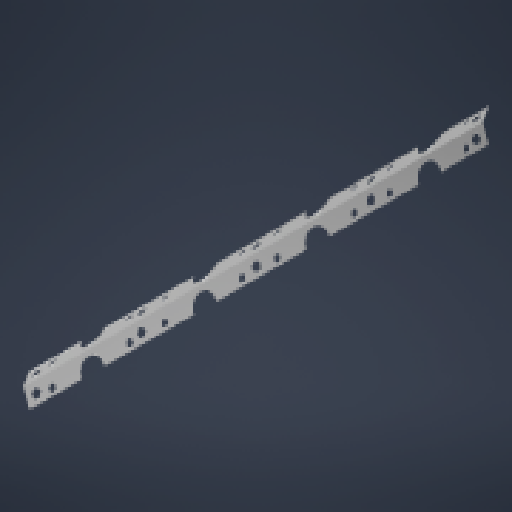
# Autodesk Inventor part: DMF 01 17 опора крышки v2.1
Saved by Autodesk Inventor 2026.2 (Build 302298010, 298A)
## iProperties
Created: 2024-04-30
Part Number: DMF 01 17 опора крышки v2.1
Material: Stainless Steel AISI 304
Document SubType Name: Sheet Metal
Designer: pokla
Density: 8 g/cm^3
Appearance: Chrome - Satin
Sheet Metal Rule: Default
Flat Pattern Width: 7.47819 cm
Flat Pattern Length: 98 cm
Flat Pattern Area: 732.863 cm^2
Sheet Metal Width: 74,782 mm
Sheet Metal Length: 980,000 mm
Sheet Metal Area: 73286,308 mm^2
Stock Number: Барабан_Полка_Крышки
Author: pokla
Autodesk Inventor part; units mm, degrees
ref_plane "YZ Plane" through (0, 0, 0) normal (1, 0, 0) x (0, 1, 0)
ref_plane "XZ Plane" through (0, 0, 0) normal (0, 1, 0) x (-1, 0, 0)
ref_plane "XY Plane" through (0, 0, 0) normal (0, 0, 1) x (1, 0, 0)
sketch "Sketch4" plane through (0, 0, 0) normal (0, 0, 1) x (1, 0, 0)
  line L0 (-196.316601, 196.316601) -> (0, 277.633599) construction
  line L1 (0, 277.633599) -> (196.316601, 196.316601) construction
  line L2 (196.316601, 196.316601) -> (277.633599, 0) construction
  line L3 (277.633599, 0) -> (196.316601, -196.316601) construction
  line L4 (196.316601, -196.316601) -> (0, -277.633599) construction
  line L5 (0, -277.633599) -> (-196.316601, -196.316601) construction
  line L6 (-196.316601, -196.316601) -> (-277.633599, 0) construction
  line L7 (-277.633599, 0) -> (-196.316601, 196.316601) construction
  line L8 (-276.999549, 1.530734) -> (-263.123447, 35.030606)
  line L9 (-276.999549, -1.530734) -> (-263.123447, -35.030606)
  arc A0 (-276.999549, 1.530734) -> (-276.999549, -1.530734) centre (-273.304031, 0) ccw
  point P0 (0, 0)
  point P1 (0, 0)
  point P2 (0, 0)
  dimension "d16" = 513
  dimension "d23" = 36.26
  dimension "d24" = 4
  measures "d16" distance between parallel lines of L7 L3
  measures "d23" distance of L8.start L8.end
  measures "d24" radius of A0
contour flange "Contour Flange1" sketch "Sketch4" thickness 2 bend radius 2 width 980 along (0, 0, -1) mid plane no both sides no wall seen from (-270.061498, 18.28067, 0) lies toward (0.9238795, -0.3826834, 0) curves L8 A0 L9
bend "Bend2"
corner "Corner2"
sketch "Эскиз14" plane through (-276.999549, 1.530734, -980) normal (-0.9238795, 0.3826834, 0) x (0, 0, 1)
  circle A0 centre (42.5, 24.403) radius 7
  line L0 (0, 36.26) -> (0, 0) projected
  line L1 (980, 36.26) -> (0, 36.26) projected
  circle A1 centre (207.5, 24.403) radius 7
  line L2 (100, 36.26) -> (100, 34.26)
  arc A2 (100, 34.26) -> (150, 34.26) centre (125, 34.26) ccw
  line L3 (150, 34.26) -> (150, 36.26)
  line L4 (42.5, 24.403) -> (207.5, 24.403) construction
  point P0 (125, 24.403)
  dimension "d100" = 14
  dimension "d101" = 42.5
  dimension "d102" = 11.857
  dimension "d103" = 165
  dimension "d104" = 14
  dimension "d135" = 2
  dimension "d136" = 25
  constraints: 6 end point, 3 centre point, 2 horizontal alignment, 2 point on circle, 2 point on line, 2 tangent, 1 horizontal, 1 midpoint, 1 perpendicular, 1 vertical, 1 vertical alignment
  measures "d100" diameter of A0
  measures "d101" distance from line of L0 L4.start
  measures "d102" distance from line of L1 L4.start
  measures "d103" distance of L4.end L4.start
  measures "d104" diameter of A1
  measures "d135" distance from line of L1 A2.centre
  measures "d136" radius of A2
extrude "Выдавливание8" cut sketch "Эскиз14" against normal through all
pattern_linear "Прямоуг.массив7" count 4 spacing 240 along (0, 0, 1) of "Выдавливание8"
sketch "Sketch6" plane through (-276.999549, 1.530734, 0) normal (-0.9238795, 0.3826834, 0) x (0.3826834, 0.9238795, 0)
  circle A0 centre (19.22, 20) radius 5.5 construction
  circle A1 centre (19.22, 960) radius 5.5 construction
  line L0 (0, 0) -> (0, 980)
  line L1 (36.26, 980) -> (0, 980)
  line L2 (36.26, 0) -> (0, 0)
  line L3 (27.62, 955.150258) -> (19.22, 950.300515)
  line L4 (19.22, 950.300515) -> (10.82, 955.150258)
  line L5 (10.82, 955.150258) -> (10.82, 964.849742)
  line L6 (10.82, 964.849742) -> (19.22, 969.699485)
  line L7 (19.22, 969.699485) -> (27.62, 964.849742)
  line L8 (27.62, 964.849742) -> (27.62, 955.150258)
  line L9 (27.62, 15.150258) -> (19.22, 10.300515)
  line L10 (19.22, 10.300515) -> (10.82, 15.150258)
  line L11 (10.82, 15.150258) -> (10.82, 24.849742)
  line L12 (10.82, 24.849742) -> (19.22, 29.699485)
  line L13 (19.22, 29.699485) -> (27.62, 24.849742)
  line L14 (27.62, 24.849742) -> (27.62, 15.150258)
  circle A2 centre (19.22, 735) radius 5.5 construction
  line L15 (27.62, 730.150258) -> (19.22, 725.300515)
  line L16 (19.22, 725.300515) -> (10.82, 730.150258)
  line L17 (10.82, 730.150258) -> (10.82, 739.849742)
  line L18 (10.82, 739.849742) -> (19.22, 744.699485)
  line L19 (19.22, 744.699485) -> (27.62, 739.849742)
  line L20 (27.62, 739.849742) -> (27.62, 730.150258)
  circle A3 centre (19.22, 490) radius 5.5 construction
  line L21 (27.62, 485.150258) -> (19.22, 480.300515)
  line L22 (19.22, 480.300515) -> (10.82, 485.150258)
  line L23 (10.82, 485.150258) -> (10.82, 494.849742)
  line L24 (10.82, 494.849742) -> (19.22, 499.699485)
  line L25 (19.22, 499.699485) -> (27.62, 494.849742)
  line L26 (27.62, 494.849742) -> (27.62, 485.150258)
  circle A4 centre (19.22, 245) radius 5.5 construction
  line L27 (27.62, 240.150258) -> (19.22, 235.300515)
  line L28 (19.22, 235.300515) -> (10.82, 240.150258)
  line L29 (10.82, 240.150258) -> (10.82, 249.849742)
  line L30 (10.82, 249.849742) -> (19.22, 254.699485)
  line L31 (19.22, 254.699485) -> (27.62, 249.849742)
  line L32 (27.62, 249.849742) -> (27.62, 240.150258)
  circle A5 centre (24.403, 772.5) radius 7
  circle A6 centre (24.403, 697.5) radius 7
  line L33 (36.26, 0) -> (36.26, 980)
  point P0 (104.588924, 0)
  dimension "d36" = 11
  dimension "d41" = 11
  dimension "d93" = 19.22
  dimension "d95" = 19.22
  dimension "d98" = 16.8
  dimension "d99" = 16.8
  dimension "d120" = 20
  dimension "d121" = 20
  dimension "d122" = 11
  dimension "d123" = 16.8
  dimension "d125" = 11
  dimension "d126" = 16.8
  dimension "d128" = 11
  dimension "d129" = 16.8
  dimension "d131" = 225
  dimension "d132" = 245
  dimension "d133" = 245
  constraints: 60 end point, 5 centre point, 5 coincident, 5 parallel, 3 vertical alignment, 65 other
  measures "d36" diameter of A0
  measures "d41" diameter of A1
  measures "d93" distance from line of L0 A0.centre
  measures "d95" distance from line of L0 A1.centre
  measures "d98" distance between parallel lines of L6 L3
  measures "d99" distance between parallel lines of L12 L9
  measures "d120" distance from line of L1 A1.centre
  measures "d121" distance from line of L2 point (19.22, 20)
  measures "d122" diameter of A2
  measures "d123" distance between parallel lines of L18 L15
  measures "d125" diameter of A3
  measures "d126" distance between parallel lines of L24 L21
  measures "d128" diameter of A4
  measures "d129" distance between parallel lines of L30 L27
  measures "d131" distance of A2.centre point (19.22, 960)
  measures "d132" distance of A3.centre A2.centre
  measures "d133" distance of A4.centre A3.centre
extrude "Extrusion1" cut sketch "Sketch6" against normal up to surface (2 mm away) contours L3 L4 L5 L6 L7 L8 | L9 L10 L11 L12 L13 L14 | L15 L16 L17 L18 L19 L20 | L21 L22 L23 L24 L25 L26 | L27 L28 L29 L30 L31 L32
mirror "Зеркальное отражение3" about plane through (0, 0, 0) normal (0, 1, 0) of "Extrusion1", "Выдавливание8", "Прямоуг.массив7"
equation "\"d16\" = Барабан_размер_по_плоскостям - Thickness"
equation "\"d24\" = BendRadius + Thickness"
equation "\"d104\" = d100"
equation "\"d41\" = d36"
equation "\"d95\" = d93"
equation "\"d99\" = d98"
equation "\"d122\" = d124"
equation "\"d125\" = d127"
equation "\"d128\" = d130"
equation "\"d25\" = Thickness"
equation "\"d26\" = BendReliefWidth"
equation "\"d27\" = BendReliefDepth"
equation "\"d28\" = MinimumRemnant"
equation "\"d29\" = TransitionRadius"
equation "\"d31\" = BendRadius"
equation "\"d33\" = CornerReliefSize"
equation "\"d34\" = GapSize"
equation "\"d35\" = JacobiRadiusSize"
equation "\"BendRadius\" = Thickness"
equation "\"BendReliefWidth\" = Thickness"
equation "\"BendReliefDepth\" = 0.5 * Thickness"
equation "\"CornerReliefSize\" = 4 * Thickness"
equation "\"MinimumRemnant\" = 2 * Thickness"
equation "\"TransitionRadius\" = BendRadius"
equation "\"JacobiRadiusSize\" = BendRadius"
equation "\"GapSize\" = Thickness"
equation "\"Барабан_размер_по_плоскостям\" = 515"
equation "\"Thickness\" = 2"
equation "\"d124\" = 11"
equation "\"d127\" = 11"
equation "\"d130\" = 11"
body "Solid2"
